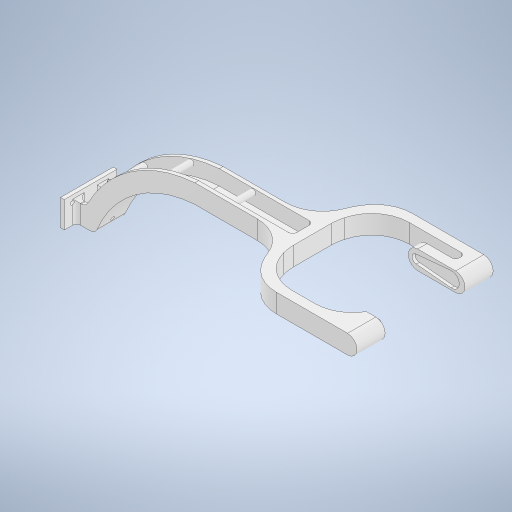
# Autodesk Inventor part: ausleger
Saved by Autodesk Inventor 2023 (Build 270158000, 158)
## iProperties
Created: 2022-06-30
Part Number: ausleger
Material: FormLabs Resin
Document SubType Name: Modeling
Designer: dennis
Density: 1.06 g/cm^3
Appearance: Smooth - White(1)
Author: dennis
Autodesk Inventor part; units mm, degrees
ref_plane "YZ Plane" through (0, 0, 0) normal (1, 0, 0) x (0, 1, 0)
ref_plane "XZ Plane" through (0, 0, 0) normal (0, 1, 0) x (-1, 0, 0)
ref_plane "XY Plane" through (0, 0, 0) normal (0, 0, 1) x (1, 0, 0)
sketch "Skizze1" plane through (0, 0, 0) normal (0, 1, 0) x (-1, 0, 0)
  line L0 (-5, -31.2505) -> (-46.177801, -31.2505)
  line L1 (-46.177801, 31.2505) -> (-5, 31.2505)
  line L2 (0, 36.2505) -> (-50, 36.2505)
  line L3 (-50, -36.2505) -> (0, -36.2505)
  line L4 (-5, 31.2505) -> (0, 31.2505)
  line L5 (-5, -31.2505) -> (0, -31.2505)
  line L6 (-51.177801, 0.024217) -> (-51.177801, 0.024217)
  line L7 (-170, -8) -> (-170, 8)
  line L8 (-190, 10) -> (-190, -10)
  line L9 (-172, 8) -> (-188, 8)
  line L10 (-188, 8) -> (-188, -8)
  line L11 (-188, -8) -> (-172, -8)
  line L12 (-172, -8) -> (-172, 8)
  line L13 (-188, -8) -> (-188, -10)
  line L14 (-188, 8) -> (-188, 10)
  line L15 (-172, 8) -> (-172, 10)
  line L16 (-172, -8) -> (-172, -10)
  line L17 (0, -21.2505) -> (0, -11.2505)
  line L18 (0, -21.2505) -> (-5, -21.2505)
  line L19 (0, 31.2505) -> (0, 21.2505)
  line L20 (0, 21.2505) -> (-5, 21.2505)
  line L21 (-5, 21.2505) -> (-10, 21.2505)
  line L22 (-10, 21.2505) -> (-10, 31.2505)
  line L23 (-5, -21.2505) -> (-10, -21.2505)
  line L24 (-10, -21.2505) -> (-10, -31.2505)
  line L25 (-10, 26.2505) -> (-30, 26.2505)
  line L26 (-30, 26.2505) -> (-30, 21.2505)
  line L27 (-30, 21.2505) -> (-10, 21.2505)
  line L28 (-30, 26.2505) -> (-30, 31.2505)
  line L29 (-170, 8) -> (-85, 8)
  line L30 (-170, -8) -> (-85, -8)
  line L31 (0, -21.2505) -> (0, 21.2505)
  line L32 (0, -36.2505) -> (0, -21.2505)
  line L33 (0, 36.2505) -> (0, 31.2505)
  line L34 (-87.378724, -10) -> (-172, -10)
  line L35 (-87.378724, 10) -> (-172, 10)
  line L36 (-188, 10) -> (-172, 10)
  line L37 (-190, 10) -> (-188, 10)
  line L38 (-190, -10) -> (-188, -10)
  line L39 (-172, -10) -> (-188, -10)
  line L40 (-50, 31.2505) -> (-46.177801, 31.2505)
  line L41 (-50, -36.2505) -> (-50, -31.2505)
  line L42 (-50, -31.2505) -> (-46.177801, -31.2505)
  line L43 (-85, -10) -> (-87.378724, -10)
  line L44 (-85, 10) -> (-87.378724, 10)
  line L45 (0, 0) -> (-60, 0)
  line L46 (-60, -10) -> (-60, 10)
  arc A0 (-50, 31.2505) -> (-60, 10) centre (-30.021258, 8.870825) ccw
  arc A1 (-60, -10) -> (-50, -31.2505) centre (-30.021258, -8.870825) ccw
  line L47 (-60, -10) -> (-65, -10)
  arc A2 (-65, -10) -> (-50, -36.2505) centre (-35.001206, -10.269041) ccw
  line L48 (-65, -10) -> (-85, -10)
  line L49 (-60, 10) -> (-65, 10)
  line L50 (-65, 10) -> (-85, 10)
  line L51 (-65, -10) -> (-65, 10)
  line L52 (-85, -8) -> (-65, -8)
  line L53 (-85, 8) -> (-65, 8)
  arc A3 (-50, 36.2505) -> (-65, 10) centre (-35.001206, 10.269041) ccw
  point P0 (-190, 0)
  point P1 (-10, 31.2505)
  point P2 (-85, 0)
  point P3 (-170, 0)
  point P4 (0, 0)
  point P5 (0, -31.2505)
  point P6 (0, -21.2505)
  dimension "d4" = 5
  dimension "d67" = 10
  dimension "d68" = 5
  dimension "d69" = 5
  dimension "d70" = 20
  dimension "d75" = 2
  dimension "d82" = 20
  dimension "d131" = 42.501
  dimension "d133" = 50
  dimension "d134" = 50
  dimension "d185" = 60
  dimension "d186" = 30
  dimension "d187" = 30
  dimension "d188" = 5
  dimension "d189" = 30
  dimension "d190" = 5
  dimension "d191" = 30
  dimension "d193" = 190
  constraints: 108 end point, 9 perpendicular, 8 horizontal, 8 parallel, 8 point on circle, 7 point on line, 5 collinear, 4 centre point, 4 midpoint, 3 vertical
  measures "d4" distance between parallel lines of L1 L2
  measures "d67" distance of L4.end L19.end
  measures "d68" distance of L20.end L21.end
  measures "d69" distance of L18.end L23.end
  measures "d70" distance of L25.start L25.end
  measures "d75" distance of L9.start L7.end
  measures "d82" distance of point (-190, 0) point (-170, 0)
  measures "d131" distance of L31.start L31.end
  measures "d133" distance of L2.start L2.end
  measures "d134" distance of L3.end L3.start
  measures "d185" distance of L45.start L45.end
  measures "d186" radius of A0
  measures "d187" radius of A1
  measures "d188" distance of L46.start L47.end
  measures "d189" radius of A2
  measures "d190" distance of L46.end L49.end
  measures "d191" radius of A3
  measures "d193" distance of L45.start point (-190, 0)
sketch "Skizze2" plane through (0, 0, 0) normal (0, 0, 1) x (1, 0, 0)
  line L0 (0, 5) -> (0, 5)
  line L1 (0, 0) -> (75, 0)
  line L2 (75, 0) -> (75, 10)
  line L3 (160, 0) -> (160, 10)
  line L4 (160, 0) -> (178, 0)
  line L5 (178, 0) -> (178, 10)
  line L6 (178, 10) -> (160, 10)
  line L7 (5, 10) -> (25.2, 10)
  line L8 (75, 10) -> (115, 10)
  line L9 (115, 10) -> (115, 0)
  line L10 (115, 0) -> (75, 0)
  line L11 (115, 10) -> (160, 10)
  line L12 (160, 0) -> (115, 0)
  line L13 (178, -40) -> (178, -30)
  line L14 (170.766577, -40) -> (178, -40)
  arc A0 (167.055742, -37.493218) -> (115, 0) centre (111.393212, -59.891494) ccw
  arc A1 (171.931442, -27.826804) -> (115, 10) centre (109.658022, -59.795869) ccw
  line L15 (175.489923, -30) -> (178, -30)
  arc A2 (171.931442, -27.826804) -> (175.489923, -30) centre (175.489923, -26) ccw
  arc A3 (167.055742, -37.493218) -> (170.766577, -40) centre (170.766577, -36) ccw
  line L16 (5, 0) -> (0, 0)
  arc A4 (5, 10) -> (0, 5) centre (5, 5) ccw
  arc A5 (0, 5) -> (5, 0) centre (5, 5) ccw
  line L17 (5, 10) -> (0, 10)
  line L18 (0, 0) -> (0, 10)
  circle A6 centre (7, 5) radius 4
  circle A7 centre (25.9, 5) radius 2.3
  line L19 (25.9, 2.7) -> (7.361783, 1.016395)
  line L20 (25.9, 7.3) -> (7.361783, 8.983605)
  circle A8 centre (7, 5) radius 1.475
  line L21 (28.2, 5) -> (30.2, 5)
  line L22 (30.2, 5) -> (30.2, 5)
  line L23 (30.2, 5) -> (30.2, 5)
  line L24 (30.2, 10) -> (5, 10)
  line L25 (25.2, 0) -> (5, 0)
  arc A9 (30.2, 5) -> (25.2, 10) centre (25.2, 5) ccw
  arc A10 (25.2, 0) -> (30.2, 5) centre (25.2, 5) ccw
  line L26 (30.2, 0) -> (30.2, 10)
  circle A11 centre (154.688887, -8.453533) radius 1.5
  circle A12 centre (168.454384, -25.188059) radius 1.5
  circle A13 centre (97.105341, 8.213516) radius 1.5
  circle A14 centre (129.991965, 5.379443) radius 1.5
  line L27 (0, 0) -> (65, 0)
  line L28 (65, 0) -> (65, 10)
  line L29 (65, 10) -> (75, 10)
  point P0 (168, -40)
  point P1 (173, -30)
  point P2 (146.051072, 0)
  point P3 (129.611578, 7.3)
  dimension "d13" = 10
  dimension "d80" = 10
  dimension "d83" = 18
  dimension "d84" = 10
  dimension "d85" = 40
  dimension "d89" = 40
  dimension "d100" = 60
  dimension "d101" = 70
  dimension "d102" = 4
  dimension "d103" = 4
  dimension "d104" = 30
  dimension "d107" = 5
  dimension "d122" = 8
  dimension "d128" = 2.95
  dimension "d141" = 2
  dimension "d142" = 5
  dimension "d178" = 3
  dimension "d179" = 3
  dimension "d182" = 3
  dimension "d183" = 3
  dimension "d192" = 65
  dimension "d194" = 178
  constraints: 60 end point, 24 point on circle, 17 tangent, 15 centre point, 15 point on line, 7 perpendicular, 6 horizontal, 3 collinear, 3 parallel, 2 concentric, 1 coincident, 1 vertical
  measures "d13" distance of L1.start L17.end
  measures "d80" distance of L1.end L2.end
  measures "d83" distance of L3.start L4.end
  measures "d84" distance of L4.end L5.end
  measures "d85" distance of L4.end L13.start
  measures "d89" distance of L2.end L8.end
  measures "d100" radius of A0
  measures "d101" radius of A1
  measures "d102" radius of A2
  measures "d103" radius of A3
  measures "d104" distance of L13.end L4.end
  measures "d107" radius of A4
  measures "d122" diameter of A6
  measures "d128" diameter of A8
  measures "d141" distance of L21.start L21.end
  measures "d142" radius of A9
  measures "d178" diameter of A11
  measures "d179" diameter of A12
  measures "d182" diameter of A13
  measures "d183" diameter of A14
  measures "d192" distance of L1.start L27.end
  measures "d194" distance of L5.end L17.end
sketch "Skizze3" plane through (0, 0, 0) normal (1, 0, 0) x (0, 1, 0)
  line L0 (-40, 14) -> (-26, 14)
  line L1 (-40, -14) -> (-40, 14)
  line L2 (-40, -14) -> (-26, -14)
  line L3 (-26, 14) -> (-26, -14)
  circle A0 centre (-29.6, 9.8) radius 1
  circle A1 centre (-35.8, 0) radius 1
  circle A2 centre (-29.6, -9.8) radius 1
  circle A3 centre (-29.6, -9.8) radius 1.8
  circle A4 centre (-35.8, 0) radius 1.8
  circle A5 centre (-29.6, 9.8) radius 1.8
  point P0 (0, 0)
  dimension "d169" = 2
  dimension "d170" = 2
  dimension "d171" = 2
  dimension "d172" = 3.6
  dimension "d173" = 3.6
  dimension "d174" = 3.6
  constraints: 8 end point, 6 centre point, 3 coincident
  measures "d169" diameter of A0
  measures "d170" diameter of A1
  measures "d171" diameter of A2
  measures "d172" diameter of A3
  measures "d173" diameter of A4
  measures "d174" diameter of A5
extrude "Extrusion5" add sketch "Skizze1" along normal blind 10 contours L5 L32 L3 L41 L42 L0 | L0 L24 L23 L18 L32 L5 | L41 A2 L47 A1 | L47 L51 L49 L46 | L20 L21 L22 L1 L4 L19 | L49 A3 L2 L33 L4 L1 L40 A0 | L27 L26 L25 L22
extrude "Extrusion6" add sketch "Skizze2" along normal mid plane 15 contours L28 L29 L2 L1 | L2 L8 L9 L10 | L9 A1 L12 | L12 A1 A2 L15 L13 L14 A3 A0 | A11 | A12 | A13 | A14
extrude "Extrusion10" add sketch "Skizze2" along normal blind 3.5 from surface at -21.2505 contours A8
draft "Flächenverjüngung1" angle 1 pull direction (0, 0, 1) faces at (8.455899, 4.763393, -18.917167) fixed edges at (5.525, 5, -21.2505)
extrude "Extrusion12" add sketch "Skizze3" along normal blind 2 from surface at 178 contours L0 L3 L2 L1 | A0 | A1 | A2 | A3 | A4 | A5
shell "Wandung2" thickness 2 removed faces 4 at (174.060242, -29.735774, 2.5) at (176.326616, -30, 2.5) at (170.305619, -24.840626, -2.5) at (98.333333, 10, 2.5)
extrude "Extrusion14" add sketch "Skizze1" along normal blind 10 contours L5 L32 L3 L41 L42 L0 | L0 L24 L23 L18 L32 L5 | L41 A2 L47 A1 | L47 L51 L49 L46 | L20 L21 L22 L1 L4 L19 | L49 A3 L2 L33 L4 L1 L40 A0 | L27 L26 L25 L22
extrude "Extrusion15" cut sketch "Skizze2" along normal mid plane 75 contours L18 A5 L1 | L18 L17 A4
extrude "Extrusion16" cut sketch "Skizze2" along normal blind 1.6 from surface at 21.2505 contours A6 | A6 L20 A7 L19 | A7 | A8
extrude "Extrusion17" cut sketch "Skizze2" along normal up to surface (5 mm away) from surface at 21.2505 contours A10 L26 L1 | A9 L24 L26
fillet "Rundung2" radius 20 9 edges at (50, 5, 36.2505) (50, 5, 31.2505) (50, 5, -31.2505) (50, 5, -36.2505) (65, 5, 7.5) (65, 5, 10) (65, 5, -7.5) (65, 5, -10) (10, 5, -31.2505)
extrude "Extrusion18" cut sketch "Skizze3" against normal up to surface from surface at 180 contours A0 | A1 | A2 round surface about axis through (111.393212, -59.891494, 0) along (0, 0, 1) radius 60 far side no
fillet "Rundung3" radius 2 10 edges at (178, -35, 7.5) (178, -34, 5.5) (178, -30, 6.5) (178, -30, -6.5) (178, -34, -5.5) (178, -35, -7.5) (65, 6, 5.5) (65, 6, -5.5) (10, 5, 26.2505) (10, 5, 31.2505)
extrude "Extrusion19" add sketch "Skizze2" along normal mid plane 15 contours A11 | A12 | A13 | A14
move or copy body "Move Body1" bodies to move or copy 1 copy no rotation origin (0, 0, 0) rotation axis (0, 1, 0) rotation angle -180 translate (86.030158, 0, 72.501)
move or copy body "Move Body2" bodies to move or copy 1 copy no translate (10, 0, -72.5)
